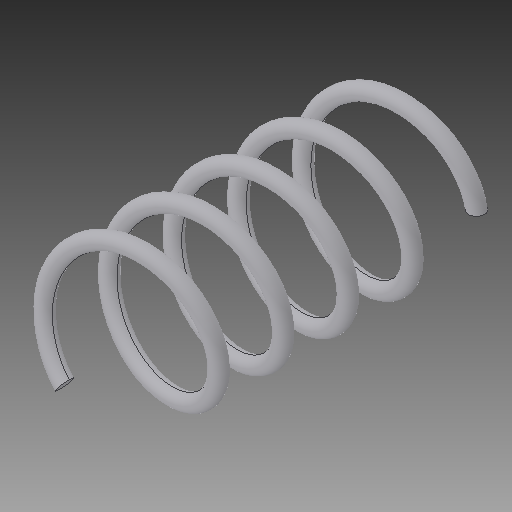
# Autodesk Inventor part: Ressort
Saved by Autodesk Inventor 2017 (Build 210142000, 142)
## iProperties
Company: FABLAB Frenchmakers
Part Number: Ressort
Material: ----------
Document SubType Name: Modeling
Designer: FABLAB Frenchmakers
Density: 7.86 g/cm^3
Appearance: Métal - Acier
Mass: 0.0980719 g
Surface Area: 1.00746 cm^2
Volume: 0.0124773 cm^3
Project: 1420 Vauban 3D XL
Catalog Web Link: http://frenchmakers.com/
Stock Number: 1420-05-18
Autodesk Inventor part; units mm, degrees
ref_plane "YZ Plane" through (0, 0, 0) normal (1, 0, 0) x (0, 1, 0)
sketch "Esquisse2" plane through (0, 0, 0) normal (0, 0, 1) x (1, 0, 0)
  circle A0 centre (0, -0.25) radius 2.067 construction
  point P0 (0, 0)
  dimension "Decalage" = 0.25
  measures "Decalage" distance of A0.centre point (0, 0)
ref_plane "Plan de construction1" through (0, 0.25, 0) normal (0, 1, 0) x (-1, 0, 0)
sketch "Esquisse3" plane through (0, 0.25, 0) normal (0, 1, 0) x (-1, 0, 0)
  line L0 (2.25, 9.3) -> (-2.25, 9.3) projected
  line L1 (2.425, 0) -> (-2.425, 0) projected
  line L2 (-2.425, 0) -> (-2.425, 5.8)
  circle A0 centre (-2.175, 0.25) radius 0.25
  line L3 (0, 0) -> (0, 9.3)
  dimension "Longueur_ressort" = 9.3
  dimension "d3" = 0.5
  constraints: 4 end point, 2 tangent, 1 centre point, 1 midpoint, 1 vertical, 1 other
  measures "Longueur_ressort" distance between parallel lines of L0 L1
  measures "d3" diameter of A0
coil "Hélicoïde1" sketch "Esquisse3" operation add axis through (0, 0.25, 0) along (0, 0, 1) pitch 2 turns 4.65 hand right contours A0
ref_plane "Plan de construction2" through (0, 0, 9.8) normal (0, 0, 1) x (1, 0, 0)
equation "\"d5\" = Longueur_ressort"
equation "\"d1\" = Decalage"
